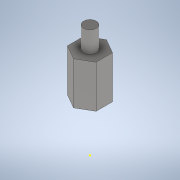
# Autodesk Inventor part: pcBOBAstandoff
Saved by Autodesk Inventor 2022 (Build 260153000, 153)
## iProperties
Created: 2021-04-30
Part Number: pcBOBAstandoff
Material: Stainless Steel
Document SubType Name: Modeling
Designer: Bowen O'Steen
Density: 8 g/cm^3
Appearance: Semi-Polished
Author: Bowen O'Steen
Autodesk Inventor part; units mm, degrees
ref_plane "YZ Plane" through (0, 0, 0) normal (1, 0, 0) x (0, 1, 0)
ref_plane "XZ Plane" through (0, 0, 0) normal (0, 1, 0) x (-1, 0, 0)
ref_plane "XY Plane" through (0, 0, 0) normal (0, 0, 1) x (1, 0, 0)
sketch "Sketch1" plane through (0, 0, 0) normal (0, 1, 0) x (-1, 0, 0)
  line L0 (3.2, 1.8475) -> (3.2, -1.8475)
  line L1 (3.2, -1.8475) -> (0, -3.695)
  line L2 (0, -3.695) -> (-3.2, -1.8475)
  line L3 (-3.2, -1.8475) -> (-3.2, 1.8475)
  line L4 (-3.2, 1.8475) -> (0, 3.695)
  line L5 (0, 3.695) -> (3.2, 1.8475)
  point P0 (0, 0)
  point P1 (3.2, 0)
  point P2 (-3.2, 0)
  dimension "d0" = 6.4
  dimension "d1" = 120
  dimension "d2" = 6.4
  constraints: 12 end point, 4 parallel, 2 horizontal alignment, 2 midpoint, 2 vertical alignment, 1 vertical
  measures "d0" distance between parallel lines of L3 L0
  measures "d1" angle of L5 L4
  measures "d2" distance between parallel lines of L2 L5
extrude "Extrusion1" add sketch "Sketch1" along normal blind 11.96
sketch "Sketch2" plane through (0, 11.96, 0) normal (0, 1, 0) x (1, 0, 0)
  circle A0 centre (0, 0) radius 1.4224
  dimension "d5" = 2.8448
  constraints: 1 centre point, 1 coincident
  measures "d5" diameter of A0
extrude "Extrusion2" add sketch "Sketch2" along normal blind 4.75
sketch "Sketch3" plane through (0, 0, 0) normal (0, -1, 0) x (1, 0, 0)
  circle A0 centre (0, 0) radius 1.4224
  dimension "d8" = 2.8448
  constraints: 1 centre point, 1 coincident
  measures "d8" diameter of A0
extrude "Extrusion3" cut sketch "Sketch3" against normal blind 6.35
sketch "Sketch4" plane through (0, 0, 0) normal (0, -1, 0) x (1, 0, 0)
  circle A0 centre (0, 0) radius 1.4224 projected
  line L0 (-3.2, -1.8475) -> (-3.2, 1.8475) projected
  line L1 (0, -3.695) -> (-3.2, -1.8475) projected
  line L2 (3.2, -1.8475) -> (0, -3.695) projected
  line L3 (3.2, 1.8475) -> (3.2, -1.8475) projected
  line L4 (0, 3.695) -> (3.2, 1.8475) projected
  line L5 (-3.2, 1.8475) -> (0, 3.695) projected
extrude "Extrusion4" add sketch "Sketch4" along normal blind 8.6233
sketch "Sketch5" plane through (0, 6.35, 0) normal (0, -1, 0) x (1, 0, 0)
  circle A0 centre (0, 0) radius 1.4224 projected
extrude "Extrusion5" add sketch "Sketch5" along normal blind 8.6233
sketch "Sketch6" plane through (0, -8.6233, 0) normal (0, -1, 0) x (1, 0, 0)
  point P0 (0, 0)
sketch "Sketch7" plane through (0, -8.6233, 0) normal (0, -1, 0) x (1, 0, 0)
  line L0 (0, -3.695) -> (3.2, -1.8475) projected
  line L1 (3.2, -1.8475) -> (3.2, 1.8475) projected
  line L2 (3.2, 1.8475) -> (0, 3.695) projected
  line L3 (0, 3.695) -> (-3.2, 1.8475) projected
  line L4 (-3.2, 1.8475) -> (-3.2, -1.8475) projected
  line L5 (-3.2, -1.8475) -> (0, -3.695) projected
  circle A0 centre (0, 0) radius 1.4224 projected
extrude "Extrusion6" cut sketch "Sketch7" against normal blind 10
sketch "Sketch8" plane through (0, -2.2733, 0) normal (0, -1, 0) x (1, 0, 0)
  circle A0 centre (0, 0) radius 1.4224 projected
extrude "Extrusion7" cut sketch "Sketch8" against normal blind 9.817
sketch "Sketch9" plane through (0, 1.3767, 0) normal (0, -1, 0) x (1, 0, 0)
  line L0 (3.2, 1.8475) -> (3.2, -1.8475) projected
  line L1 (0, 3.695) -> (3.2, 1.8475) projected
  line L2 (-3.2, 1.8475) -> (0, 3.695) projected
  line L3 (-3.2, -1.8475) -> (-3.2, 1.8475) projected
  line L4 (0, -3.695) -> (-3.2, -1.8475) projected
  line L5 (3.2, -1.8475) -> (0, -3.695) projected
  circle A0 centre (0, 0) radius 1.4224 projected
  circle A1 centre (0, 0) radius 1.4224 projected
extrude "Extrusion8" cut sketch "Sketch9" against normal blind 1.058
sketch "Sketch10" plane through (0, 7.5437, 0) normal (0, -1, 0) x (1, 0, 0)
  circle A0 centre (0, 0) radius 1.4224 projected
extrude "Extrusion9" cut sketch "Sketch10" against normal blind 1.058
body "Solid1"
